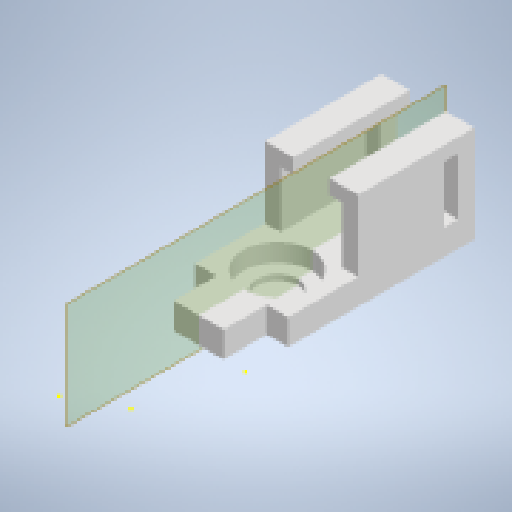
# Autodesk Inventor part: techo
Saved by Autodesk Inventor 2023 (Build 270158000, 158)
## iProperties
Created: 2024-07-31
Part Number: techo
Material: Generic
Document SubType Name: Sheet Metal
Designer: sebas
Density: 1 g/cm^3
Sheet Metal Rule: Default_mm
Appearance: Default
Author: sebas
Autodesk Inventor part; units mm, degrees
ref_plane "YZ Plane" through (0, 0, 0) normal (1, 0, 0) x (0, 1, 0)
ref_plane "XZ Plane" through (0, 0, 0) normal (0, 1, 0) x (-1, 0, 0)
ref_plane "XY Plane" through (0, 0, 0) normal (0, 0, 1) x (1, 0, 0)
sketch "Sketch1" plane through (0, 0, 0) normal (0, 1, 0) x (-1, 0, 0)
  line L0 (0, 0) -> (65, 0)
  line L1 (65, 0) -> (65, -200)
  line L2 (65, -200) -> (0, -200)
  line L3 (0, -200) -> (0, 0)
  dimension "d0" = 65
  dimension "d1" = 200
  constraints: 8 end point, 3 perpendicular, 1 horizontal
  measures "d0" distance of L0.start L0.end
  measures "d1" distance of L0.end L1.end
extrude "Extrusion1" add sketch "Sketch1" along normal blind 18
sketch "Sketch2" plane through (0, 18, 0) normal (0, 1, 0) x (1, 0, 0)
  line L0 (0, 0) -> (0, 200) projected
  line L1 (0, 0) -> (-32.5, 0)
  line L2 (-65, 0) -> (0, 0) projected
  line L3 (-32.5, 0) -> (-32.5, 8)
  line L4 (-32.5, 8) -> (-55.5, 8)
  line L5 (-55.5, 8) -> (-55.5, 18.5)
  line L6 (-55.5, 18.5) -> (-9.5, 18.5)
  line L7 (-9.5, 18.5) -> (-9.5, 8)
  line L8 (-9.5, 8) -> (-32.5, 8)
  dimension "d4" = 8
  dimension "d5" = 23
  dimension "d6" = 10.5
  dimension "d7" = 46
  dimension "d8" = 10.5
  constraints: 14 end point, 3 perpendicular, 1 horizontal, 1 midpoint, 1 point on line
  measures "d4" distance of L1.end L3.end
  measures "d5" distance of L3.end L4.end
  measures "d6" distance of L4.end L5.end
  measures "d7" distance of L5.end L6.end
  measures "d8" distance of L6.end L7.end
extrude "Extrusion2" cut sketch "Sketch2" against normal through all
sketch "Sketch3" plane through (0, 18, 0) normal (0, 1, 0) x (1, 0, 0)
  line L0 (-55.5, 18.5) -> (-9.5, 18.5) projected
  line L1 (-32.5, 18.5) -> (-32.5, 135)
  circle A0 centre (-32.5, 135) radius 23.75
  point P0 (0, 0)
  dimension "d11" = 116.5
  dimension "d12" = 47.5
  constraints: 2 end point, 1 centre point, 1 coincident, 1 midpoint, 1 vertical
  measures "d11" distance of L1.start L1.end
  measures "d12" diameter of A0
extrude "Extrusion3" cut sketch "Sketch3" against normal blind 12.5
sketch "Sketch4" plane through (-32.5, 5.5, -135) normal (0, 1, 0) x (1, 0, 0)
  circle A0 centre (0, 0) radius 14
  point P0 (32.5, -135)
  dimension "d15" = 28
  constraints: 1 centre point
  measures "d15" diameter of A0
extrude "Extrusion4" cut sketch "Sketch4" against normal blind 4
sketch "Sketch7" plane through (0, 18, 0) normal (0, 1, 0) x (1, 0, 0)
  line L0 (0, 200) -> (-65, 200) projected
  line L1 (-65, 200) -> (0, 200)
  line L2 (-32.5, 200) -> (-32.5, 158.75)
  circle A0 centre (-32.5, 135) radius 23.75 projected
  line L3 (-32.5, 200) -> (-11, 200)
  line L4 (-11, 200) -> (-54, 200)
  line L5 (0, 0) -> (0, 200) projected
  line L6 (-11, 200) -> (-11, 158.75)
  line L7 (-54, 200) -> (-54, 158.75)
  line L8 (-54, 158.75) -> (-65, 158.75)
  line L9 (-65, 200) -> (-65, 0) projected
  line L10 (-65, 200) -> (-54, 200)
  line L11 (-11, 158.75) -> (0, 158.75)
  line L12 (0, 200) -> (0, 158.75)
  line L13 (0, 200) -> (-11, 200)
  dimension "d19" = 21.5
  dimension "d20" = 43
  constraints: 22 end point, 5 point on line, 2 horizontal, 2 parallel, 1 collinear, 1 midpoint, 1 perpendicular, 1 vertical, 1 vertical alignment, 1 other
  measures "d19" distance of L2.start L3.end
  measures "d20" distance of L3.end L4.end
extrude "Extrusion5" add sketch "Sketch7" along normal blind 39.5 contours L5 L11 L6 L0 | L7 L8 L9 L0
sketch "Sketch8" plane through (0, 57.5, 0) normal (0, 1, 0) x (1, 0, 0)
  line L0 (0, 0) -> (0, 200) projected
  line L1 (-11, 200) -> (-54, 200) projected
  line L2 (0, 200) -> (-11, 200)
  line L3 (0, 200) -> (-65, 200) projected
  line L4 (-11, 200) -> (-20, 200)
  line L5 (-20, 200) -> (-20, 158.75)
  line L6 (-20, 158.75) -> (0, 158.75)
  line L7 (0, 200) -> (0, 158.75)
  line L8 (-65, 158.75) -> (-54.25, 158.75)
  line L9 (-54.25, 158.75) -> (-45.25, 158.75)
  line L10 (-45.25, 158.75) -> (-45.25, 200)
  line L11 (-54, 200) -> (-65, 200) projected
  line L12 (-65, 200) -> (-45.25, 200)
  line L13 (-65, 159.6209) -> (-65, 200)
  line L14 (-65, 200) -> (-65, 158.75) projected
  line L15 (-65, 200) -> (-65, 158.75)
  dimension "d23" = 9
  dimension "d24" = 9
  constraints: 22 end point, 4 collinear, 4 point on line, 3 perpendicular, 1 horizontal
  measures "d23" distance of L1.start L4.end
  measures "d24" distance of L8.end L9.end
extrude "Extrusion6" add sketch "Sketch8" along normal blind 10
sketch "Sketch10" plane through (0, 0, -200) normal (0, 0, -1) x (-1, 0, 0)
  line L0 (20, 57.5) -> (11, 57.5) projected
  line L1 (20, 57.5) -> (20, 67.5) projected
  line L2 (20, 57.5) -> (20, 67.5)
  line L3 (20, 67.5) -> (0, 67.5) projected
  line L4 (20, 67.5) -> (0, 67.5)
  line L5 (0, 67.5) -> (0, 0)
  line L6 (0, 0) -> (65, 0) projected
  line L7 (0, 0) -> (65, 0)
  line L8 (65, 0) -> (65, 67.5) projected
  line L9 (65, 0) -> (65, 67.5)
  line L10 (45.25, 67.5) -> (65, 67.5) projected
  line L11 (65, 67.5) -> (45.25, 67.5)
  line L12 (45.25, 57.5) -> (45.25, 67.5) projected
  line L13 (45.25, 67.5) -> (45.25, 57.5)
  line L14 (45.25, 57.5) -> (54, 57.5) projected
  line L15 (45.25, 57.5) -> (54, 57.5)
  line L16 (54, 18) -> (54, 57.5) projected
  line L17 (54, 57.5) -> (54, 18)
  line L18 (11, 18) -> (11, 57.5) projected
  line L19 (54, 18) -> (11, 18)
  line L20 (11, 18) -> (11, 57.5)
  line L21 (11, 57.5) -> (20, 57.5)
  constraints: 24 end point, 7 perpendicular, 5 collinear
extrude "Extrusion7" add sketch "Sketch10" along normal blind 40
sketch "Sketch14" plane through (0, 0, 0) normal (1, 0, 0) x (0, 0, -1)
  line L0 (240, 67.5) -> (240, 57.5) projected
  line L1 (240, 67.5) -> (228.3141, 67.5)
  line L2 (158.75, 67.5) -> (240, 67.5) projected
  line L3 (228.3141, 67.5) -> (228.3141, 18)
  line L4 (240, 18) -> (158.75, 18) projected
  line L5 (228.3141, 18) -> (218.3141, 18)
  line L6 (218.3141, 18) -> (218.3141, 67.5)
  line L7 (218.3141, 67.5) -> (228.3141, 67.5)
  line L8 (218.3141, 67.5) -> (218.3141, 57.5)
  line L9 (218.3141, 57.5) -> (228.3141, 57.5)
  line L10 (158.75, 57.5) -> (240, 57.5) projected
  point P0 (0, 0)
  dimension "d29" = 10
  constraints: 14 end point, 6 point on line, 4 perpendicular
  measures "d29" distance of L3.end L5.end
extrude "Extrusion8" cut sketch "Sketch14" against normal through all contours L3 L4 L6 L9
sketch "Sketch17" plane through (0, 18, 0) normal (0, 1, 0) x (1, 0, 0)
  line L0 (0, 158.75) -> (0, 240) projected
  line L1 (0, 240) -> (0, 110)
  line L2 (0, 0) -> (0, 240) projected
  line L3 (0, 110) -> (0, 90)
  line L4 (0, 90) -> (-15, 90)
  line L5 (-65, 0) -> (-65, 240) projected
  line L6 (-15, 90) -> (-15, 110)
  line L7 (-15, 110) -> (0, 110)
  line L8 (-15, 90) -> (-15, 80)
  line L9 (-65, 80) -> (-65, 110)
  line L10 (-65, 110) -> (-50, 110)
  line L11 (-50, 110) -> (-50, 80)
  line L12 (-50, 80) -> (-15, 80)
  line L13 (-65, 80) -> (-65, 0)
  line L14 (-65, 0) -> (0, 0) projected
  line L15 (0, 0) -> (0, 110)
  dimension "d33" = 130
  dimension "d34" = 20
  dimension "d35" = 15
  dimension "d36" = 10
  dimension "d37" = 15
  dimension "d38" = 30
  constraints: 24 end point, 5 perpendicular, 5 point on line, 2 collinear, 1 horizontal
  measures "d33" distance of L0.end L1.end
  measures "d34" distance of L1.end L3.end
  measures "d35" distance of L3.end L4.end
  measures "d36" distance of L4.end L8.end
  measures "d37" distance of L9.end L10.end
  measures "d38" distance of L10.end L11.end
extrude "Extrusion9" cut sketch "Sketch17" against normal through all
sketch "Sketch18" plane through (-50, 18, -80) normal (0, 0, 1) x (1, 0, 0)
  point P0 (50, -18)
sketch "Sketch19" plane through (0, 18, 0) normal (0, 1, 0) x (1, 0, 0)
  point P0 (0, 0)
sketch "Sketch20" plane through (-50, 18, -110) normal (-1, 0, 0) x (0, 0, 1)
  point P0 (110, -18)
sketch "Sketch21" plane through (0, 18, 0) normal (0, 1, 0) x (1, 0, 0)
  point P0 (0, 0)
ref_plane "Work Plane1" through (-32.5, 18, -158.75) normal (-1, 0, 0) x (0, 0, 1)
ref_plane "Work Plane2" through (-32.5, 18, -158.75) normal (1, 0, 0) x (0, 0, -1)
equation "\"BendRadius\" = Thickness"
equation "\"BendReliefWidth\" = Thickness"
equation "\"BendReliefDepth\" = 0.5 * Thickness"
equation "\"CornerReliefSize\" = 4 * Thickness"
equation "\"MinimumRemnant\" = 2 * Thickness"
equation "\"TransitionRadius\" = BendRadius"
equation "\"JacobiRadiusSize\" = BendRadius"
equation "\"GapSize\" = Thickness"
equation "\"Thickness\" = 0.5"
body "Solid1"
